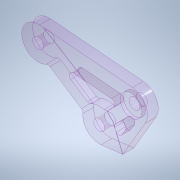
# Autodesk Inventor part: 後ろウィング中間挟むフレームver2
Saved by Autodesk Inventor 2020.2 (Build 242310000, 310)
## iProperties
Created: 2020-05-07
Part Number: 後ろウィング中間挟むフレームver2
Material: ポリカーボネート、クリア
Document SubType Name: Modeling
Designer: mozar
Density: 1.2 g/cm^3
Appearance: ポリカーボネート - クリア
Mass: 1.2825 g
Surface Area: 12.7384 cm^2
Volume: 1.06875 cm^3
Author: mozar
Autodesk Inventor part; units mm, degrees
ref_plane "YZ Plane" through (0, 0, 0) normal (1, 0, 0) x (0, 1, 0)
ref_plane "XZ Plane" through (0, 0, 0) normal (0, 1, 0) x (-1, 0, 0)
ref_plane "XY Plane" through (0, 0, 0) normal (0, 0, 1) x (1, 0, 0)
sketch "スケッチ1" plane through (0, 0, 0) normal (0, 0, 1) x (1, 0, 0)
  line L0 (-101.5, 47.999998) -> (108.5, 47.999998)
  circle A0 centre (111.885049, -39.000002) radius 4
  circle A1 centre (191.876682, -37.842982) radius 4
  circle A2 centre (111.885049, -39.000002) radius 7
  circle A3 centre (191.876682, -37.842982) radius 7
  line L1 (191.876682, -37.842982) -> (111.885049, -39.000002) construction
  line L2 (191.775442, -30.843714) -> (111.78381, -32.000734)
  line L3 (111.986288, -45.99927) -> (191.977921, -44.84225)
  arc A4 (191.977921, -44.84225) -> (191.775442, -30.843714) centre (191.876682, -37.842982) ccw
  arc A5 (111.78381, -32.000734) -> (111.986288, -45.99927) centre (111.885049, -39.000002) ccw
  line L4 (193.542302, -31.044032) -> (241.704818, -42.842982)
  circle A6 centre (234.566446, -71.981335) radius 30
  line L5 (262.587356, -82.697145) -> (213.725294, -50.402494)
  line L6 (213.725294, -50.402494) -> (190.211062, -44.641931)
  line L7 (264.566446, -121.542906) -> (264.566446, -63.2267)
  line L8 (111.885049, -39.000002) -> (111.885049, 40.999998) construction
  line L9 (118.885049, -39.000002) -> (118.885049, 40.999998)
  line L10 (104.885049, 40.999998) -> (104.885049, -39.000002)
  arc A7 (104.885049, -39.000002) -> (118.885049, -39.000002) centre (111.885049, -39.000002) ccw
  arc A8 (118.885049, 40.999998) -> (104.885049, 40.999998) centre (111.885049, 40.999998) ccw
  circle A9 centre (58.238326, 51.481995) radius 30
  line L11 (113.558078, 34.202868) -> (65.408448, 22.351438)
  line L12 (28.441083, 47.999998) -> (86.70408, 42.010942)
  line L13 (86.70408, 42.010942) -> (110.21202, 47.797128)
  circle A10 centre (113.5, -20.000002) radius 68
  line L14 (315.327237, -100.585467) -> (70.600424, 104.764712)
  line L15 (253.850074, -49.000002) -> (111.885049, -39.000002)
  arc A11 (93.592427, -27.104845) -> (135.370976, -5.924402) centre (95.060351, 21.794105) ccw
  arc A12 (135.370976, -5.924402) -> (135.847591, -3.671647) centre (132.898992, -4.224609) ccw
  arc A13 (135.847591, -3.671647) -> (83.183341, 18.55647) centre (102.157897, -9.989602) ccw
  line L16 (111.885049, -39.000002) -> (112.74718, 40.995353) construction
  line L17 (118.884642, -39.075438) -> (119.746773, 40.919916)
  line L18 (105.747586, 41.070789) -> (104.885455, -38.924565)
  arc A14 (104.885455, -38.924565) -> (118.884642, -39.075438) centre (111.885049, -39.000002) ccw
  arc A15 (119.746773, 40.919916) -> (105.747586, 41.070789) centre (112.74718, 40.995353) ccw
  line L19 (164.994898, 47.999998) -> (164.994898, 25.999998)
  line L20 (164.994898, 25.999998) -> (327.494898, -102.000002)
  circle A16 centre (116.292557, -40.000002) radius 68
  circle A17 centre (-98.885049, -0.000002) radius 67.5
  line L21 (321.363327, -8.500986) -> (-152.668056, 78.49822)
  line L22 (104.889695, -3) -> (104.889695, 0)
  line L23 (104.889695, -3) -> (64.444342, -3)
  line L24 (72.06562, 0) -> (104.889695, 0)
  circle A18 centre (83.376901, -17.5) radius 13.85
  line L25 (198.510163, -35.607603) -> (190.779084, -12.665641)
  line L26 (185.2432, -40.07836) -> (169.408184, 6.912016)
  circle A19 centre (197.837392, 16.492211) radius 30
  line L27 (190.779084, -12.665641) -> (191.876682, 45.89408)
  circle A20 centre (191.876682, -37.842982) radius 83.737062
  line L28 (191.876682, 45.89408) -> (191.876682, -37.842982)
  line L29 (96.889695, -3) -> (96.889695, -6)
  line L30 (96.889695, -6) -> (87.889695, -6)
  line L31 (87.889695, -6) -> (87.889695, -3)
  line L32 (76.444342, -3) -> (76.444342, -6)
  line L33 (76.444342, -6) -> (67.444342, -6)
  line L34 (67.444342, -6) -> (67.444342, -3)
  line L35 (99.889695, -3) -> (99.889695, 0)
  line L36 (99.889695, 0) -> (84.889695, 0)
  line L37 (84.889695, 0) -> (84.889695, -3)
  line L38 (79.444342, -3) -> (79.444342, 0)
  line L39 (79.444342, 0) -> (64.444342, 0)
  line L40 (64.444342, 0) -> (64.444342, -3)
  line L41 (64.444342, 0) -> (59.444342, 0)
  line L42 (59.444342, 0) -> (59.444342, -3)
  line L43 (59.444342, -3) -> (64.444342, -3)
  line L44 (59.444342, -3) -> (59.444342, -6)
  circle A21 centre (111.885049, -39.000002) radius 1.5
  circle A22 centre (111.885049, -39.000002) radius 9
  circle A23 centre (111.885049, -39.000002) radius 10
  circle A24 centre (111.885049, -39.000002) radius 15
  line L45 (121.057661, -50.868582) -> (142.927269, -50.552254)
  line L46 (121.057661, -50.868582) -> (127.651316, -45.772687)
  line L47 (127.651316, -45.772687) -> (126.808053, -37.482129)
  line L48 (124.15135, -30.366471) -> (104.889695, -3)
  line L49 (101.060181, -49.383751) -> (59.444342, -6)
  circle A25 centre (95.889695, -6) radius 1
  circle A26 centre (88.889695, -6) radius 1
  circle A27 centre (95.889695, -3) radius 1
  circle A28 centre (88.889695, -3) radius 1
  circle A29 centre (100.889695, -3) radius 1
  circle A30 centre (83.889695, -3) radius 1
  circle A31 centre (80.444342, -3) radius 1
  circle A32 centre (75.444342, -6) radius 1
  circle A33 centre (68.444342, -6) radius 1
  circle A34 centre (75.444342, -3) radius 1
  circle A35 centre (68.444342, -3) radius 1
  circle A36 centre (63.444342, -3) radius 1
  line L50 (189.021336, -49.498324) -> (211.692496, -55.05235)
  line L51 (211.692496, -55.05235) -> (259.830429, -86.868398)
  circle A37 centre (191.876682, -37.842982) radius 8
  circle A38 centre (191.876682, -37.842982) radius 13
  line L52 (198.876682, -21.280236) -> (198.876682, -52.125839)
  circle A39 centre (194.376682, -52.125839) radius 4.5
  circle A40 centre (194.376682, -52.125839) radius 1.5
  circle A41 centre (177.559162, -35.549813) radius 1.5
  circle A42 centre (194.376682, -52.125839) radius 4.5
  circle A43 centre (177.559162, -35.549813) radius 4.5
  circle A44 centre (191.876682, -37.842982) radius 1.5
  circle A45 centre (191.876682, -37.842982) radius 4.5
  line L53 (198.809292, -51.349976) -> (196.309292, -37.06712)
  line L54 (192.588355, -33.399613) -> (178.270835, -31.106444)
  circle A46 centre (181.698047, -48.169907) radius 1.5
  circle A47 centre (181.698047, -48.169907) radius 4.5
  line L55 (193.03634, -56.42159) -> (180.357706, -52.465659)
  line L56 (177.422129, -49.572237) -> (173.283244, -36.952142)
  point P0 (0, 0)
  point P1 (0, 0)
  point P2 (0, 0)
  point P3 (151.880865, -38.421492)
  point P4 (111.885049, 0.999998)
  point P5 (105.885049, -0.000002)
  point P6 (105.885049, -0.000002)
  point P7 (23.732778, -42.728965)
  point P8 (112.316114, 0.997675)
  point P9 (76.444342, -4.5)
  point P10 (99.889695, -1.5)
  point P11 (74.444342, -6)
  point P12 (69.444342, -6)
  point P13 (69.444342, -3)
  point P14 (74.444342, -3)
  point P15 (82.889695, -3)
  point P16 (81.444342, -3)
  point P17 (62.444342, -3)
  point P18 (101.889695, -3)
  point P19 (89.889695, -3)
  point P20 (94.889695, -3)
  point P21 (94.889695, -6)
  point P22 (89.889695, -6)
  point P23 (118.961603, -31.934425)
  point P24 (118.924491, -31.897449)
  point P25 (118.962007, -31.896907)
  point P26 (119.12697, -45.895985)
  point P27 (104.885049, -3)
  point P28 (104.885049, -31.858573)
  point P29 (117.642551, -45.917456)
  point P30 (175.94693, -45.074126)
  point P31 (193.036341, -56.421591)
  point P32 (198.871572, -51.911454)
  point P33 (198.876682, -51.912706)
  point P34 (198.876682, -46.764852)
  point P35 (193.972807, -45.563491)
  point P36 (184.006402, -36.408166)
  point P37 (182.178049, -30.982533)
  point P38 (117.440072, -31.91892)
  point P39 (180.360015, -43.873438)
  point P40 (180.33295, -43.821464)
  point P41 (180.497374, -43.833046)
  point P42 (180.545532, -31.470772)
  point P43 (180.516681, -31.522351)
  point P44 (180.526062, -31.467653)
  point P45 (193.972807, -45.563491)
  point P46 (197.96776, -46.542182)
  point P47 (197.449702, -43.582445)
  point P48 (186.057217, -32.353552)
  point P49 (182.445104, -31.775017)
  point P50 (184.006402, -36.408166)
  dimension "d27" = 167.47412
  dimension "d62" = 9
  dimension "d0" = 8
  dimension "d1" = 8
  dimension "d2" = 3
  dimension "d3" = 3
  dimension "d4" = 80
  dimension "d5" = 14
  dimension "d6" = 14
  dimension "d7" = 60
  dimension "d8" = 14
  dimension "d9" = 60
  dimension "d10" = 14
  dimension "d11" = 6
  dimension "d12" = 40
  dimension "d13" = 13.271
  dimension "d14" = 14
  dimension "d15" = 10
  dimension "d16" = 5
  dimension "d17" = 22
  dimension "d18" = 150
  dimension "d19" = 162.5
  dimension "d20" = 0
  dimension "d21" = 136
  dimension "d22" = 136
  dimension "d23" = 135
  dimension "d24" = 38.2272
  dimension "d25" = 25
  dimension "d26" = 60
  dimension "d28" = 5
  dimension "d29" = 3
  dimension "d30" = 5
  dimension "d31" = 3
  dimension "d32" = 3
  dimension "d33" = 5
  dimension "d34" = 1
  dimension "d35" = 5
  dimension "d36" = 5
  dimension "d37" = 2
  dimension "d38" = 2
  dimension "d39" = 2
  dimension "d40" = 2
  dimension "d41" = 2
  dimension "d42" = 2
  dimension "d43" = 2
  dimension "d44" = 2
  dimension "d45" = 2
  dimension "d46" = 2
  dimension "d47" = 2
  dimension "d48" = 2
  dimension "d49" = 5
  dimension "d50" = 1
  dimension "d51" = 6
  dimension "d52" = 3
  dimension "d53" = 3
  dimension "d54" = 3
  dimension "d55" = 3
  dimension "d56" = 3
  dimension "d57" = 3
  dimension "d58" = 109.028
  dimension "d59" = 3
  dimension "d60" = 9
  dimension "d61" = 72.2057
  dimension "d63" = 54.514
  constraints: 118 end point, 59 tangent, 46 centre point, 45 point on circle, 16 vertical, 8 coincident, 8 point on line, 7 equal length, 7 horizontal, 5 midpoint, 5 parallel, 1 concentric, 1 perpendicular, 1 vertical alignment, 29 other
  measures "d0" diameter of A0
  measures "d1" diameter of A1
  measures "d2" radial gap between concentric circles of A0 A2
  measures "d3" radial gap between concentric circles of A1 A3
  measures "d4" distance of L1.start L1.end
  measures "d5" diameter of A5
  measures "d6" distance from line of L4 L5.end
  measures "d7" diameter of A6
  measures "d8" diameter of A8
  measures "d9" diameter of A9
  measures "d10" distance from line of L11 L12.end
  measures "d11" horizontal distance of L1.end point (105.885, 0)
  measures "d12" angle of L14 L0
  measures "d14" diameter of A15
  measures "d15" vertical distance of L15.start L1.end
  measures "d16" vertical distance of L1.start L4.end
  measures "d17" distance of L19.start L19.end
  measures "d18" vertical distance of L19.start L20.end
  measures "d19" distance from line of L19 L20.end
  measures "d20" distance from line of L19.start L0
  measures "d21" diameter of A10
  measures "d22" diameter of A16
  measures "d23" diameter of A17
  measures "d24" angle of L0 L20
  measures "d25" distance from line of L5.start L20
  measures "d26" diameter of A19
  measures "d28" distance between parallel lines of L35 L22
  measures "d29" distance of L41.end L42.end
  measures "d30" distance of L42.end L40.end
  measures "d31" distance of L42.end L44.end
  measures "d32" diameter of A21
  measures "d33" radial gap between concentric circles of A0 A22
  measures "d34" radial gap between concentric circles of A22 A23
  measures "d35" radial gap between concentric circles of A23 A24
  measures "d36" distance between parallel lines of L3 L45
  measures "d37" diameter of A25
  measures "d38" diameter of A26
  measures "d39" diameter of A27
  measures "d40" diameter of A28
  measures "d41" diameter of A29
  measures "d42" diameter of A30
  measures "d43" diameter of A31
  measures "d44" diameter of A32
  measures "d45" diameter of A33
  measures "d46" diameter of A34
  measures "d47" diameter of A35
  measures "d48" diameter of A36
  measures "d49" distance between parallel lines of L6 L50
  measures "d50" radial gap between concentric circles of A3 A37
  measures "d51" radial gap between concentric circles of A3 A38
  measures "d52" diameter of A40
  measures "d53" diameter of A41
  measures "d54" radial gap between concentric circles of A40 A42
  measures "d55" radial gap between concentric circles of A41 A43
  measures "d56" diameter of A44
  measures "d57" radial gap between concentric circles of A44 A45
  measures "d59" diameter of A46
  measures "d60" diameter of A47
  measures "d61" angle of L26 L2
extrude "押し出し1" add sketch "スケッチ1" against normal blind 3 contours L56 L3 A10 | A10 L3 A47 L56 | L55 A47 A16 | A16 A47 A38 A39 L55 | A10 L15 A38 A47 L3 | L3 L56 L15 A10 | A47 L3 A38 A16 | A16 A38 A47 | A39 A38 L50 A40 L52 | A47 A38 L3 | L15 L56 A43 A10 | A10 A43 A38 L15 | A38 L3 A16 | A16 L3 A47 A38 | A47 L3 A37 L6 L53 A38 A39 | A39 L50 A38 | L50 A40 A38 A39 | A38 A47 L15 A16 L3 | A38 L15 A47 | A43 A38 A10 | A10 A38 A43 | A38 A43 A10 L54 L26 A37 A16 L15 A47 | A16 A47 L3 | A38 A40 L50 | L50 A39 A38 | A39 A38 L53 | A47 L15 | A38 A43 A10 | A10 A43 A38 | A47 A16 L15 A37 L3 | A47 L15 A16 | A43 A38 A10 | L54 A10 A38 A43 | A37 L15 A3 L6 L3 | L3 L6 A37 | A16 A37 L15 | L6 A37 L15 L53 | L6 A3 L3 | L3 A3 L15 A37 L6 | A37 A16 L26 A3 L15 | A37 L26 A16 | L15 A37 L53 | A3 L15 | A3 L54 L28 A45 L53 L15 | L15 A3 L53 A37 | A37 A16 L26 | L26 L54 A16 A37 | L26 A16 A37 L54 A3 | A16 L54 A37 | A45 | L54 A45 L28 | A1
extrude "押し出し2" cut sketch "スケッチ1" against normal blind 0.05 contours A37 L15 A3 L6 L3 | L3 L6 A37 | L6 A37 L15 L53 | L6 A3 L3 | L3 A3 L15 A37 L6 | A37 A16 L26 A3 L15 | A37 L26 A16 | L15 A37 L53 | L52 A37 | A37 L53 A3 L52 | A3 L15 | A3 L54 L28 A45 L53 L15 | L15 A3 L53 A37 | A37 A16 L26 | L26 L54 A16 A37 | A37 L52 A3 L25 L4 | L4 L25 A37 | A3 L53 A45 L54 L28 | L26 A16 A37 L54 A3 | A16 L54 A37 | L25 A3 L4 | L4 A3 L28 A37 L25 | L28 A3 L2 A37 | L2 A3 L54 A37 | A3 L28 L54 | A45 | L54 A45 L28 | A1 | A44
sketch "スケッチ2" plane through (0, 0, 0) normal (0, 0, 1) x (1, 0, 0)
  circle A0 centre (181.698047, -48.169907) radius 1.5
  circle A1 centre (177.559162, -35.549813) radius 1.5
  circle A2 centre (194.376682, -52.125839) radius 1.5
  line L0 (197.96776, -46.542182) -> (193.972807, -45.563491)
  arc A3 (184.006402, -36.408166) -> (193.972807, -45.563491) centre (191.876682, -37.842982) ccw
  line L1 (184.006402, -36.408166) -> (182.445104, -31.775017)
  line L2 (182.445104, -31.775017) -> (180.545532, -31.470772)
  arc A4 (180.545532, -31.470772) -> (180.516681, -31.522351) centre (191.876682, -37.842982) ccw
  arc A5 (180.516681, -31.522351) -> (180.526062, -31.467653) centre (113.5, -20.000002) ccw
  line L3 (180.526062, -31.467653) -> (178.270835, -31.106444)
  arc A6 (178.270835, -31.106444) -> (173.283244, -36.952142) centre (177.559162, -35.549813) ccw
  line L4 (173.283244, -36.952142) -> (177.422129, -49.572237)
  arc A7 (177.422129, -49.572237) -> (180.357706, -52.465659) centre (181.698047, -48.169907) ccw
  line L5 (180.357706, -52.465659) -> (193.03634, -56.42159)
  arc A8 (193.03634, -56.42159) -> (198.809292, -51.349976) centre (194.376682, -52.125839) ccw
  line L6 (198.809292, -51.349976) -> (197.96776, -46.542182)
  circle A9 centre (191.876682, -37.842982) radius 1.5
  circle A10 centre (191.876682, -37.842982) radius 3
  point P0 (0, 0)
  dimension "d68" = 6
  constraints: 1 centre point, 1 coincident
  measures "d68" diameter of A10
extrude "押し出し3" cut sketch "スケッチ2" against normal blind 1 contours A10
sketch "スケッチ3" plane through (0, 0, 0) normal (0, 0, 1) x (1, 0, 0)
  line L0 (194.745121, -45.752694) -> (213.725294, -50.402494)
  line L1 (213.725294, -50.402494) -> (262.587356, -82.697145)
  arc A0 (262.587356, -82.697145) -> (241.704818, -42.842982) centre (234.566446, -71.981335) ccw
  line L2 (241.704818, -42.842982) -> (193.542302, -31.044032)
  arc A1 (193.542302, -31.044032) -> (185.418769, -40.543975) centre (191.876682, -37.842982) ccw
  line L3 (185.418769, -40.543975) -> (191.206612, -54.382359)
  line L4 (191.206612, -54.382359) -> (195.655899, -53.216469)
  line L5 (195.655899, -53.216469) -> (195.656069, -53.216296)
  arc A2 (195.656069, -53.216296) -> (195.656308, -53.216236) centre (194.922022, -50.307486) ccw
  line L6 (195.656308, -53.216236) -> (198.568436, -51.556289)
  line L7 (198.568436, -51.556289) -> (199.758723, -49.040078)
  line L8 (199.758723, -49.040078) -> (195.762722, -50.087189)
  arc A3 (194.586681, -49.505705) -> (195.762722, -50.087189) centre (195.50924, -49.119849) ccw
  line L9 (194.586681, -49.505705) -> (193.584616, -47.109828)
  arc A4 (194.745121, -45.752694) -> (193.584616, -47.109828) centre (194.507175, -46.723972) ccw
  circle A5 centre (191.876682, -37.842982) radius 4.025
  circle A6 centre (111.885049, -39.000002) radius 4.025
  line L10 (182.178049, -30.982533) -> (117.440072, -31.91892)
  arc A7 (117.440072, -31.91892) -> (117.642551, -45.917456) centre (111.885049, -39.000002) ccw
  line L11 (117.642551, -45.917456) -> (175.94693, -45.074126)
  line L12 (175.94693, -45.074126) -> (177.422132, -49.57224)
  arc A8 (177.422132, -49.57224) -> (180.357708, -52.465661) centre (181.698049, -48.169909) ccw
  line L13 (180.357708, -52.465661) -> (193.036341, -56.42159)
  arc A9 (193.036341, -56.42159) -> (198.871572, -51.911454) centre (194.376682, -52.125838) ccw
  line L14 (198.871572, -51.911454) -> (198.876682, -51.912706)
  line L15 (198.876682, -51.912706) -> (198.876682, -46.764852)
  line L16 (198.876682, -46.764852) -> (193.972807, -45.563491)
  arc A10 (184.006402, -36.408166) -> (193.972807, -45.563491) centre (191.876682, -37.842982) ccw
  line L17 (184.006402, -36.408166) -> (182.178049, -30.982533)
  circle A11 centre (194.376682, -52.125839) radius 1.5
  circle A12 centre (177.559161, -35.549813) radius 1.5
  circle A13 centre (181.698049, -48.169909) radius 1.5
  arc A14 (180.497374, -43.833046) -> (180.360015, -43.873438) centre (181.698049, -48.169909) ccw
  arc A15 (180.33295, -43.821464) -> (180.360015, -43.873438) centre (191.876682, -37.842982) ccw
  line L18 (180.33295, -43.821464) -> (180.497374, -43.833046)
  line L19 (191.876682, -37.842982) -> (111.885049, -39.000002) construction
  line L20 (191.775442, -30.843714) -> (111.78381, -32.000734)
  line L21 (111.986288, -45.99927) -> (191.977921, -44.84225)
  arc A16 (191.977921, -44.84225) -> (191.775442, -30.843714) centre (191.876682, -37.842982) ccw
  arc A17 (111.78381, -32.000734) -> (111.986288, -45.99927) centre (111.885049, -39.000002) ccw
  circle A18 centre (178.961677, -35.529526) radius 4.5
  circle A19 centre (178.961677, -35.529526) radius 1.5
  circle A20 centre (183.157555, -46.799925) radius 1.5
  circle A21 centre (183.157555, -46.799925) radius 4.5
  line L22 (182.178049, -30.982533) -> (117.440072, -31.91892)
  line L23 (197.834841, -41.517261) -> (208.997311, -23.41636)
  line L24 (197.834841, -41.517261) -> (181.973255, -67.238185)
  circle A22 centre (170.35293, -38.154307) radius 4.5
  circle A23 centre (170.35293, -38.154307) radius 1.5
  line L25 (188.270523, -60.320544) -> (180.805974, -42.473256)
  arc A24 (194.73203, -26.18764) -> (180.805974, -42.473256) centre (191.876682, -37.842982) ccw
  line L26 (194.73203, -26.18764) -> (242.894547, -37.986589)
  arc A25 (264.570959, -90.00158) -> (242.894547, -37.986589) centre (234.566446, -71.981335) ccw
  line L27 (264.570959, -90.00158) -> (211.692496, -55.05235)
  line L28 (208.863654, -41.485411) -> (202.414104, -55.119458)
  line L29 (202.414104, -55.119458) -> (198.735697, -57.216192)
  line L30 (198.735697, -57.216192) -> (198.256714, -57.703764)
  line L31 (198.256714, -57.703764) -> (188.270523, -60.320544)
  line L32 (189.614177, -50.574943) -> (183.680676, -51.269416)
  arc A26 (184.006402, -36.408166) -> (193.972807, -45.563491) centre (191.876682, -37.842982) ccw
  point P0 (0, 0)
  point P1 (0, 0)
  point P2 (0, 0)
  point P3 (151.880865, -38.421492)
  point P4 (186.913184, -44.11703)
  point P5 (186.913184, -44.11703)
  point P6 (179.020383, -45.029671)
  point P7 (186.913184, -44.11703)
  point P8 (179.020383, -45.029671)
  dimension "d75" = 9
  dimension "d71" = 14
  dimension "d72" = 9
  dimension "d73" = 3
  dimension "d74" = 3
  dimension "d76" = 122.49
  dimension "d77" = 9
  dimension "d78" = 3
  dimension "d79" = 5
  dimension "d80" = 7
  constraints: 68 end point, 34 point on circle, 26 centre point, 7 tangent, 3 coincident, 3 point on line, 1 collinear, 1 equal radius, 1 midpoint, 1 parallel, 56 other
  measures "d71" diameter of A17
  measures "d72" diameter of A18
  measures "d73" diameter of A19
  measures "d74" diameter of A20
  measures "d76" angle of L23 L11
  measures "d77" diameter of A22
  measures "d78" diameter of A23
  measures "d79" distance between parallel lines of L3 L25
  measures "d80" distance of L32.start point (186.913, -44.117)
extrude "押し出し4" cut sketch "スケッチ3" against normal blind 10 contours L0 L24 A2 L9 A4 | A4 L9 A2 L24 L3 L21 A10 L16 | L0 L15 L8 A2 L24 | L24 L9 A2 | A2 L8 A3 L9 L24 | L9 L24 A2 | L21 L3 A10 | L15 L7 L6 A2 L8 | A2 L6 A11 L24 L9 A3 L8 | A2 A11 L4 L3 L24 | L15 L14 A9 L13 L24 L3 L4 A11 A2 L6 L7 | L24 L13 L25 L32 L3 | A2 L6 | A2 L4 A11 | L25 L13 A8 L12 L21 A21 L32 picked at (195.430042, -53.271235)
extrude "押し出し5" add sketch "スケッチ3" against normal blind 3 contours A22 | A20 A13 | A13 L25 A20 | A13 L25 | A19 A12 | A12 A19 | A23 picked at (182.922726, -47.847814)
hole "穴1" at (183.157555, -46.799925, 0) at (178.961677, -35.529526, 0) at (170.35293, -38.154307, 0) direction (0, 0, -1) diameter 3 depth 12 tip angle 118
sketch "スケッチ4" plane through (0, 0, 0) normal (0, 0, 1) x (1, 0, 0)
  circle A0 centre (191.876682, -37.842982) radius 3
  line L0 (196.309292, -37.06712) -> (197.96776, -46.542182)
  arc A1 (196.309292, -37.06712) -> (192.588355, -33.399613) centre (191.876682, -37.842982) ccw
  line L1 (182.445104, -31.775017) -> (192.588355, -33.399613)
  line L2 (184.006402, -36.408166) -> (182.445104, -31.775017)
  arc A2 (184.006402, -36.408166) -> (186.913184, -44.11703) centre (191.876682, -37.842982) ccw
  arc A3 (186.913184, -44.11703) -> (193.972807, -45.563491) centre (191.876682, -37.842982) ccw
  line L3 (197.96776, -46.542182) -> (193.972807, -45.563491)
  circle A4 centre (178.961677, -35.529526) radius 1.5
  circle A5 centre (183.157555, -46.799925) radius 1.5
  circle A6 centre (170.35293, -38.154307) radius 1.5
  line L4 (174.353347, -40.21505) -> (175.94693, -45.074126)
  line L5 (175.94693, -45.074126) -> (179.020383, -45.029671)
  arc A7 (179.020383, -45.029671) -> (183.680676, -51.269416) centre (183.157555, -46.799925) ccw
  line L6 (183.680676, -51.269416) -> (189.614177, -50.574943)
  line L7 (189.614177, -50.574943) -> (186.913184, -44.11703)
  arc A8 (184.006402, -36.408166) -> (186.913184, -44.11703) centre (191.876682, -37.842982) ccw
  line L8 (184.006402, -36.408166) -> (182.445104, -31.775017)
  line L9 (182.445104, -31.775017) -> (180.545532, -31.470772)
  arc A9 (180.545532, -31.470772) -> (180.516681, -31.522351) centre (191.876682, -37.842982) ccw
  arc A10 (180.516681, -31.522351) -> (180.526062, -31.467653) centre (113.5, -20.000002) ccw
  line L10 (180.526062, -31.467653) -> (178.270835, -31.106444)
  arc A11 (178.270835, -31.106444) -> (173.153722, -34.632153) centre (177.559162, -35.549813) ccw
  arc A12 (173.153722, -34.632153) -> (174.353347, -40.21505) centre (170.35293, -38.154307) ccw
  line L11 (179.020383, -45.029671) -> (175.94693, -45.074126)
  circle A13 centre (183.157555, -46.799925) radius 4.5
  circle A14 centre (178.961677, -35.529526) radius 4.5
  circle A15 centre (170.35293, -38.154307) radius 4.5
  circle A16 centre (191.876682, -37.842982) radius 4.5
  arc A17 (173.153722, -34.632153) -> (174.353347, -40.21505) centre (170.35293, -38.154307) ccw
  line L12 (169.040539, -33.849933) -> (177.649287, -31.225153)
  arc A18 (173.153722, -34.632153) -> (174.353347, -40.21505) centre (170.35293, -38.154307) ccw
  line L13 (180.639428, -50.529407) -> (167.834803, -41.883789)
  line L14 (189.614177, -50.574943) -> (195.75637, -40.122898)
  line L15 (192.670134, -33.413486) -> (179.755129, -31.10003)
  line L16 (182.445104, -31.775017) -> (182.37584, -31.569476)
  point P0 (0, 0)
  point P1 (174.608405, -32.152308)
  point P2 (178.196132, -31.095122)
  point P3 (192.405207, -45.825504)
  point P4 (186.913184, -44.11703)
  dimension "d92" = 9
  dimension "d93" = 9
  constraints: 10 end point, 8 point on circle, 7 tangent, 4 coincident, 3 centre point, 1 collinear, 1 point on line, 3 other
  measures "d92" diameter of A14
  measures "d93" diameter of A16
extrude "押し出し6" cut sketch "スケッチ4" against normal blind 10 contours L0 L3 A3 L14 A16 | A14 L12 A11
extrude "押し出し7" add sketch "スケッチ4" against normal blind 3 contours L1 L16 L15 | L14 L7 A3 | L9 A14 L15 L16 | L9 A9 A10 L10 A11 A14 | A7 L13 A12 L4 L5 | A11 A12 L12 picked at (179.170572, -31.203466)
extrude "押し出し8" cut sketch "スケッチ4" against normal blind 0.05 contours L1 L16 L15
extrude "押し出し9" cut sketch "スケッチ4" against normal blind 0.05 contours L14 L7 A3
sketch "スケッチ5" plane through (0, 0, 0) normal (0, 0, 1) x (1, 0, 0)
  circle A0 centre (175.744086, -41.453294) radius 1.5
  circle A1 centre (166.361389, -35.71178) radius 1.5
  circle A2 centre (111.885049, -39.000002) radius 6
  circle A3 centre (183.157555, -46.799925) radius 1.5
  line L0 (186.913184, -44.11703) -> (189.614177, -50.574943)
  line L1 (189.614177, -50.574943) -> (183.680676, -51.269416)
  arc A4 (179.020383, -45.029671) -> (183.680676, -51.269416) centre (183.157555, -46.799925) ccw
  line L2 (179.020383, -45.029671) -> (178.464745, -45.037708)
  arc A5 (173.128236, -45.114896) -> (178.464745, -45.037708) centre (175.744086, -41.453294) ccw
  line L3 (173.128236, -45.114896) -> (117.642551, -45.917456)
  arc A6 (117.440072, -31.91892) -> (117.642551, -45.917456) centre (111.885049, -39.000002) ccw
  line L4 (117.440072, -31.91892) -> (167.598953, -31.193409)
  line L5 (167.598953, -31.193409) -> (184.919442, -41.792263)
  arc A7 (184.919442, -41.792263) -> (186.913184, -44.11703) centre (191.876682, -37.842982) ccw
  arc A8 (180.33295, -43.821464) -> (180.360015, -43.873438) centre (191.876682, -37.842982) ccw
  arc A9 (180.497374, -43.833046) -> (180.360015, -43.873438) centre (181.698049, -48.169909) ccw
  line L6 (180.497374, -43.833046) -> (180.33295, -43.821464)
  line L7 (169.040539, -33.849933) -> (177.649287, -31.225153)
  arc A10 (179.755129, -31.10003) -> (177.649287, -31.225153) centre (178.961677, -35.529526) ccw
  line L8 (179.755129, -31.10003) -> (182.37584, -31.569476)
  line L9 (182.37584, -31.569476) -> (184.006402, -36.408166)
  arc A11 (184.006402, -36.408166) -> (186.913184, -44.11703) centre (191.876682, -37.842982) ccw
  line L10 (186.913184, -44.11703) -> (189.614177, -50.574943)
  line L11 (189.614177, -50.574943) -> (183.680676, -51.269416)
  arc A12 (180.639428, -50.529407) -> (183.680676, -51.269416) centre (183.157555, -46.799925) ccw
  line L12 (180.639428, -50.529407) -> (167.834803, -41.883789)
  arc A13 (169.040539, -33.849933) -> (167.834803, -41.883789) centre (170.35293, -38.154307) ccw
  circle A14 centre (178.961677, -35.529526) radius 1.5
  circle A15 centre (183.157555, -46.799925) radius 1.5
  circle A16 centre (170.35293, -38.154307) radius 1.5
  circle A17 centre (166.361389, -35.71178) radius 4.5
  circle A18 centre (191.876682, -37.842982) radius 4.5
  circle A19 centre (175.744086, -41.453294) radius 4.5
  line L13 (192.251246, -33.358597) -> (166.735953, -31.227396)
  line L14 (164.012587, -39.550156) -> (173.395285, -45.291671)
  line L15 (173.111819, -45.103112) -> (180.525289, -50.449743)
  arc A20 (195.75637, -40.122898) -> (192.670134, -33.413486) centre (191.876682, -37.842982) ccw
  line L16 (182.37584, -31.569476) -> (192.670134, -33.413486)
  line L17 (184.006402, -36.408166) -> (182.37584, -31.569476)
  arc A21 (184.006402, -36.408166) -> (186.913184, -44.11703) centre (191.876682, -37.842982) ccw
  line L18 (189.614177, -50.574943) -> (186.913184, -44.11703)
  line L19 (189.614177, -50.574943) -> (195.75637, -40.122898)
  circle A22 centre (191.876682, -37.842982) radius 3
  point P0 (0, 0)
  point P1 (0, 0)
  point P2 (170.975898, -33.259849)
  point P3 (173.249983, -45.202757)
  point P4 (167.918247, -41.94013)
  point P5 (192.670134, -33.413486)
  point P6 (175.296712, -31.942446)
  point P7 (167.799691, -31.316246)
  point P8 (168.71019, -31.873404)
  point P9 (165.964533, -37.15833)
  point P10 (167.468818, -34.700049)
  dimension "d107" = 9
  dimension "d106" = 9
  constraints: 20 end point, 18 point on circle, 12 centre point, 5 tangent, 3 coincident, 44 other
  measures "d106" diameter of A17
extrude "押し出し10" add sketch "スケッチ5" against normal blind 3 contours A14
extrude "押し出し12" add sketch "スケッチ5" against normal blind 3 contours A17 A16 | A16 A17
extrude "押し出し13" cut sketch "スケッチ5" against normal blind 10 contours L14 L3 L12 | L7 A10 L8 L9 L13 | L3 L14 L15 A4 L12 | L9 L16 A18 L13
extrude "押し出し14" add sketch "スケッチ5" against normal blind 3 contours A1 A13 A17 L7 | A13 L12 L14 A17 | A17 L5 L7 | L5 L13 L7 | A17 L13 L5
extrude "押し出し11" cut sketch "スケッチ5" against normal blind 0.05 contours L7 L13 L9 A11 L5 | L5 L13 L7 | L7 A10 L8 L9 L13 | A14
hole "穴2" at (175.744086, -41.453294, 0) at (166.361389, -35.71178, 0) direction (0, 0, -1) diameter 3 depth 12 tip angle 118
sketch "スケッチ6" plane through (0, 0, 0) normal (0, 0, 1) x (1, 0, 0)
  circle A0 centre (166.361389, -35.71178) radius 1.5
  circle A1 centre (175.744086, -41.453294) radius 1.5
  line L0 (173.249983, -45.202757) -> (164.012587, -39.550156)
  arc A2 (166.735953, -31.227396) -> (164.012587, -39.550156) centre (166.361389, -35.71178) ccw
  line L1 (166.735953, -31.227396) -> (192.251246, -33.358597)
  arc A3 (195.75637, -40.122898) -> (192.251246, -33.358597) centre (191.876682, -37.842982) ccw
  line L2 (195.75637, -40.122898) -> (189.614177, -50.574943)
  line L3 (189.614177, -50.574943) -> (183.680676, -51.269416)
  arc A4 (180.525289, -50.449743) -> (183.680676, -51.269416) centre (183.157555, -46.799925) ccw
  line L4 (180.525289, -50.449743) -> (173.249983, -45.202757)
  circle A5 centre (183.157555, -46.799925) radius 1.5
  circle A6 centre (191.876682, -37.842982) radius 1.5
  line L5 (192.001536, -36.348187) -> (166.486244, -34.216985)
  arc A7 (166.486244, -34.216985) -> (165.578455, -36.991239) centre (166.361389, -35.71178) ccw
  line L6 (165.578455, -36.991239) -> (174.912719, -42.703115)
  line L7 (174.912719, -42.703115) -> (182.280133, -48.016531)
  arc A8 (182.280133, -48.016531) -> (183.331929, -48.289755) centre (183.157555, -46.799925) ccw
  line L8 (183.331929, -48.289755) -> (187.783606, -47.768719)
  line L9 (187.783606, -47.768719) -> (193.169911, -38.602954)
  arc A9 (193.169911, -38.602954) -> (192.001536, -36.348187) centre (191.876682, -37.842982) ccw
  circle A10 centre (166.361389, -35.71178) radius 4.5
  circle A11 centre (175.744086, -41.453294) radius 4.5
  circle A12 centre (183.157555, -46.799925) radius 4.5
  circle A13 centre (191.876682, -37.842982) radius 4.5
  circle A14 centre (177.000249, -36.098665) radius 1
  circle A15 centre (175.393639, -35.964471) radius 1
  point P0 (0, 0)
  dimension "d121" = 3
  dimension "d122" = 3
  dimension "d123" = 3
  dimension "d124" = 3
  dimension "d125" = 3
  dimension "d126" = 2
  dimension "d127" = 2
  constraints: 10 end point, 9 centre point, 6 point on circle, 4 tangent, 7 other
  measures "d121" distance between parallel lines of L1 L5
  measures "d122" radial gap between concentric circles of A0 A10
  measures "d123" radial gap between concentric circles of A1 A11
  measures "d124" radial gap between concentric circles of A5 A12
  measures "d125" radial gap between concentric circles of A6 A13
  measures "d126" diameter of A14
  measures "d127" diameter of A15
sketch "スケッチ7" plane through (0, 0, 0) normal (0, 0, 1) x (1, 0, 0)
  arc A0 (187.108208, -40.591072) -> (186.474889, -38.897013) centre (186.391652, -39.893542) ccw
  line L0 (185.499908, -42.243239) -> (187.108208, -40.591072)
  arc A1 (184.487753, -42.501021) -> (185.499908, -42.243239) centre (184.783352, -41.545709) ccw
  arc A2 (184.487753, -42.501021) -> (180.939384, -42.884607) centre (183.157555, -46.799925) ccw
  arc A3 (179.895523, -42.849085) -> (180.939384, -42.884607) centre (180.446457, -42.014536) ccw
  line L1 (175.356109, -39.852349) -> (179.895523, -42.849085)
  arc A4 (175.990281, -38.021271) -> (175.356109, -39.852349) centre (175.907044, -39.0178) ccw
  line L2 (186.474889, -38.897013) -> (175.990281, -38.021271)
  arc A5 (187.538379, -45.771145) -> (189.374048, -46.049175) centre (188.511895, -45.542527) ccw
  arc A6 (187.538379, -45.771145) -> (187.419116, -45.354554) centre (183.157555, -46.799925) ccw
  arc A7 (187.649574, -44.33583) -> (187.419116, -45.354554) centre (188.36613, -45.03336) ccw
  line L3 (188.772362, -43.182418) -> (187.649574, -44.33583)
  arc A8 (190.35107, -44.386596) -> (188.772362, -43.182418) centre (189.488918, -43.879948) ccw
  line L4 (189.374048, -46.049175) -> (190.35107, -44.386596)
  arc A9 (178.68556, -46.298668) -> (183.680676, -51.269416) centre (183.157555, -46.799925) ccw
  line L5 (183.680676, -51.269416) -> (189.614177, -50.574943)
  line L6 (189.614177, -50.574943) -> (195.75637, -40.122898)
  arc A10 (195.75637, -40.122898) -> (192.251246, -33.358597) centre (191.876682, -37.842982) ccw
  line L7 (192.251246, -33.358597) -> (166.735953, -31.227396)
  arc A11 (166.735953, -31.227396) -> (168.57956, -39.627098) centre (166.361389, -35.71178) ccw
  arc A12 (169.623422, -39.662621) -> (168.57956, -39.627098) centre (169.072487, -40.497169) ccw
  line L8 (169.623422, -39.662621) -> (178.242718, -45.352729)
  arc A13 (178.68556, -46.298668) -> (178.242718, -45.352729) centre (177.691783, -46.187278) ccw
  circle A14 centre (191.876682, -37.842982) radius 1.5
  circle A15 centre (166.361389, -35.71178) radius 1.5
  circle A16 centre (183.157555, -46.799925) radius 1.5
  circle A17 centre (166.361389, -35.71178) radius 1.5
  circle A18 centre (175.744086, -41.453294) radius 1.5
  circle A19 centre (183.157555, -46.799925) radius 1.5
  line L9 (184.919442, -41.792263) -> (167.799691, -31.316246)
  line L10 (167.799691, -31.316246) -> (166.735953, -31.227396)
  arc A20 (166.735953, -31.227396) -> (164.012587, -39.550156) centre (166.361389, -35.71178) ccw
  line L11 (164.012587, -39.550156) -> (173.249983, -45.202757)
  line L12 (173.249983, -45.202757) -> (180.525289, -50.449743)
  arc A21 (180.525289, -50.449743) -> (183.680676, -51.269416) centre (183.157555, -46.799925) ccw
  line L13 (183.680676, -51.269416) -> (189.614177, -50.574943)
  line L14 (189.614177, -50.574943) -> (186.913184, -44.11703)
  arc A22 (184.919442, -41.792263) -> (186.913184, -44.11703) centre (191.876682, -37.842982) ccw
  point P0 (0, 0)
  point P1 (0, 0)
  point P2 (164.012587, -39.550156)
  point P3 (187.393343, -45.265063)
  point P4 (187.805385, -46.250231)
  constraints: 28 point on circle, 18 end point, 17 centre point, 66 other
extrude "押し出し15" cut sketch "スケッチ7" against normal blind 10 contours A11 A12 L8 A13 A9 L12 L11
extrude "押し出し16" add sketch "スケッチ7" against normal blind 3 contours A18 L1 | L1 A18
extrude "押し出し17" cut sketch "スケッチ7" against normal blind 2.5 contours L0 A1 A22 L9 L2 A0 | L9 A22 A1 A2 A3 L1 A18 A4 L2 | A7 L3 A8 L4 A5 L14 | A18 L1 picked at (176.206148, -40.331367)
equation "\"d9\" = d7"
equation "\"d26\" = d7"
equation "\"d63\" = 0.5 * d58"
